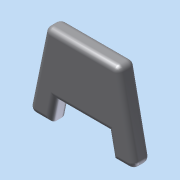
# Autodesk Inventor part: RUCBase
Saved by Autodesk Inventor 2011 SP1 (Build 150282100, 282)
## iProperties
Created: 2011-08-15
Part Number: RUCBase
Document SubType Name: Modeling
Designer: dgitz
Density: 1 g/cm^3
Author: dgitz
Autodesk Inventor part; units mm, degrees
ref_plane "YZ Plane" through (0, 0, 0) normal (1, 0, 0) x (0, 1, 0)
ref_plane "XZ Plane" through (0, 0, 0) normal (0, 1, 0) x (-1, 0, 0)
ref_plane "XY Plane" through (0, 0, 0) normal (0, 0, 1) x (1, 0, 0)
sketch "Sketch1" plane through (0, 0, 0) normal (0, 0, 1) x (1, 0, 0)
  line L0 (-21.434, 104.1719) -> (-59.534, -92.6781)
  line L1 (-59.534, -92.6781) -> (-8.734, -92.6781)
  line L2 (-8.734, -92.6781) -> (1.0982, -41.8781)
  line L3 (1.0982, -41.8781) -> (121.1337, -41.8781)
  line L4 (121.1337, -41.8781) -> (130.966, -92.6781)
  line L5 (130.966, -92.6781) -> (181.766, -92.6781)
  line L6 (181.766, -92.6781) -> (143.666, 104.1719)
  line L7 (143.666, 104.1719) -> (-21.434, 104.1719)
  point P0 (0, 0)
  dimension "d0" = 50.8
  dimension "d5" = 241.3
  dimension "d6" = 50.8
  dimension "d7" = 196.85
  dimension "d8" = 165.1
  dimension "d12" = 100.954
  dimension "d13" = 100.954
  constraints: 16 end point, 3 equal length, 3 horizontal, 3 parallel
  measures "d0" distance of L1.end L0.end
  measures "d5" distance of L5.end L0.end
  measures "d6" distance between parallel lines of L3 L1
  measures "d7" distance between parallel lines of L7 L1
  measures "d8" distance of L6.end L0.start
  measures "d12" angle of L0 L7
  measures "d13" angle of L6 L7
extrude "Extrusion1" add sketch "Sketch1" along normal blind 38.1
fillet "Fillet1" radius 12.7 20 edges at (61.116, 104.1719, 38.1) (-40.484, 5.7469, 38.1) (-34.134, -92.6781, 38.1) (-3.8179, -67.2781, 38.1) (61.116, -41.8781, 38.1) (126.0498, -67.2781, 38.1) (156.366, -92.6781, 38.1) (162.716, 5.7469, 38.1) (61.116, 104.1719, 0) (-40.484, 5.7469, 0) (-34.134, -92.6781, 0) (-3.8179, -67.2781, 0) (61.116, -41.8781, 0) (126.0498, -67.2781, 0) (156.366, -92.6781, 0) (162.716, 5.7469, 0) (143.666, 104.1719, 19.05) (181.766, -92.6781, 19.05) (-21.434, 104.1719, 19.05) (-59.534, -92.6781, 19.05)
body "Solid1"
